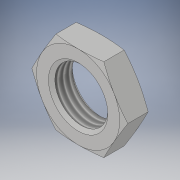
# Autodesk Inventor part: 5362901 M10x1
Saved by Autodesk Inventor 2019 (Build 230136000, 136)
## iProperties
Created: 2023-03-28
Part Number: 5362901 M10x1
Material: Generic
Catalog Web Link: www.cadenas.de
Description: DSNU-nut-nut
Vendor: FESTO
Document SubType Name: Modeling
Designer: psAdmin
Manufacturer: FESTO
Mass: 0.417855 g
Surface Area: 4.9508 cm^2
Volume: 0.417855 cm^3
Density: 1 g/cm^3
Appearance: PSOLRGB-175-175-175
Category: PARTsolutions
Company: FESTO
Title: 5362901 M10x1
Author: Cadenas PARTsolutions
Comments: nut
PSOL_IDENT_0: {$CADENAS_DATA/23d-libs/festo/parts/d/dsnu/parts/dsnu_nut.prj},168 {VTYP=3D},{NB=5362901 M10x1},{LIN
PSOL_IDENT_1: A=5362901 M10x1},{NN=DSNU-nut},{DATE=13.03.2023 13:59:39},{GEOMDATE=08.08.2018 13:11:10},{VERSION=},
PSOL_IDENT_2: {LINEID=20},{WBVAR=},{WBNUMERIC=}  {NB=5362901 M10x1},{LINA=5362901 M10x1},{KT=DUMMY},{TNR=5362901},
PSOL_IDENT_3: {TYP=M10x1},{SW=14.000},{M=10.000},{L=4.000},{KV=14.000}
NB: 5362901 M10x1
NN: DSNU-nut
NT: nut
NBSYN: $TNR. $TYP.
LINA: 5362901 M10x1
CATALOG: Festo
TNR: 5362901
TYP: M10x1
SW: 14
M: 10
L: 4
KV: 14
SUPPLIER: FESTO
ARTICLENO: 5362901 M10x1
BOMINFO: 5362901 M10x1
CREATOR: CADENAS GmbH
Autodesk Inventor part; units mm, degrees
sketch "Sketch_1" plane through (0, 0, 0) normal (0, 0, 1) x (1, 0, 0)
  line L0 (-8.0829, 0) -> (-4.0415, -7)
  line L1 (-4.0415, -7) -> (4.0415, -7)
  line L2 (4.0415, -7) -> (8.0829, 0)
  line L3 (8.0829, 0) -> (4.0415, 7)
  line L4 (4.0415, 7) -> (-4.0415, 7)
  line L5 (-4.0415, 7) -> (-8.0829, 0)
  constraints: 12 end point
extrude "Extrusion1" add sketch "Sketch_1" along normal blind 4
sketch "Sketch_2" plane through (0, 0, 0) normal (1, 0, 0) x (0, 1, 0)
  line L0 (0, 0) -> (0, 4)
  line L1 (0, 4) -> (5, 4)
  line L2 (5, 4) -> (4.4585, 3.4585)
  line L3 (4.4585, 3.4585) -> (4.4585, 0.5415)
  line L4 (4.4585, 0.5415) -> (5, 0)
  line L5 (5, 0) -> (0, 0)
  line L6 (0, 0) -> (0, 4)
  constraints: 14 end point
revolve "Revolution1" cut sketch "Sketch_2" angle 360 about axis through (0, 0, 0) along (0, 0, -1)
thread "Thread1" size "M10x1" class "6H" standard "ISO Metric profile" full length
sketch "Sketch_3" plane through (0, 0, 0) normal (1, 0, 0) x (0, 1, 0)
  line L0 (0, -50) -> (0, 50)
  line L1 (17, 4) -> (7, 4)
  line L2 (7, 4) -> (13, 2.3923)
  line L3 (13, 2.3923) -> (13, 1.6077)
  line L4 (13, 1.6077) -> (7, 0)
  line L5 (7, 0) -> (17, 0)
  line L6 (17, 0) -> (17, 4)
  constraints: 14 end point
revolve "Revolution2" cut sketch "Sketch_3" angle 360 about axis through (0, 0, -50) along (0, 0, -1)
ref_plane "ANBAU_XY" through (0, 0, 0) normal (0, 0, -1) x (1, 0, 0)
ref_plane "ANBAU_YZ" through (0, 0, 0) normal (1, 0, 0) x (0, -1, 0)
ref_plane "ANBAU_ZX" through (0, 0, 0) normal (0, -1, 0) x (0, 0, -1)
body "Solid1"
